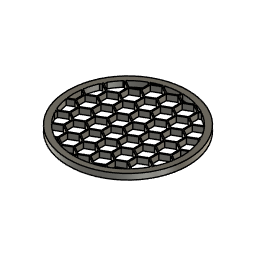
thermal_protection (Autodesk Fusion 360 design; units mm, degrees)
Autodesk Fusion 360 part; units mm, degrees
sketch "Sketch1" plane through (0, 0, 0) normal (0, 0, 1) x (1, 0, 0)
  circle A0 centre (0, 0) radius 21
  line L0 (0, -1.6166) -> (0, 1.6166)
  line L1 (0, 1.6166) -> (-2.8, 3.2332)
  line L2 (-2.8, 3.2332) -> (-5.6, 1.6166)
  line L3 (-5.6, 1.6166) -> (-5.6, -1.6166)
  line L4 (-5.6, -1.6166) -> (-2.8, -3.2332)
  line L5 (-2.8, -3.2332) -> (0, -1.6166)
  line L6 (5.6, -1.6166) -> (5.6, 1.6166)
  line L7 (5.6, 1.6166) -> (2.8, 3.2332)
  line L8 (2.8, 3.2332) -> (0, 1.6166)
  line L9 (0, 1.6166) -> (0, -1.6166)
  line L10 (0, -1.6166) -> (2.8, -3.2332)
  line L11 (2.8, -3.2332) -> (5.6, -1.6166)
  line L12 (-2.8, 0) -> (0, 0) construction
  line L13 (-2.8, 0) -> (-1.4, 2.4249) construction
  point P0 (-2.8, 0)
  point P1 (2.8, 0)
  dimension "d5" = 42
  dimension "d6" = 5.6
  constraint coincident A0.centre L12.end
  constraint vertical L3
  constraint vertical L0
  constraint coincident A0.centre L0
  constraint midpoint A0.centre L0
  constraint parallel L0 L9
  constraint coincident L0.end L1.start
  constraint coincident L0.start L5.end
  constraint coincident P0 L12.start
  constraint midpoint L1 L13.end
  measures "d5" diameter of A0
  measures "d6" distance of L0 L3
extrude "Extrude3" add sketch "Sketch1" along normal blind 2 thin wall 0.2 inside contours L0 L1 L2 L3 L4 L5 L9
extrude "Extrude4" add sketch "Sketch1" along normal up to surface (2 mm away) thin wall 0.2 inside contours L0 L6 L7 L8 L9 L10 L11
pattern_linear "R-Pattern2" count 14 spacing 5.6 along (1, 0, 0) both ways count 12 spacing 5.6 along (0.5, 0.866025, 0) both ways of "Extrude4"
extrude "Extrude5" cut sketch "Sketch1" along normal up to surface (2 mm away) contours A0 | L0 L1 L2 L3 L4 L5 L9 | L0 L6 L7 L8 L9 L10 L11 keep common part
extrude "Extrude6" add sketch "Sketch1" along normal up to surface (2 mm away) thin wall 2 inside contours A0 | L0 L1 L2 L3 L4 L5 L9 | L0 L6 L7 L8 L9 L10 L11
equation "OD = 42 mm"
equation "wall = 0.4 mm"
equation "owall = 2 mm"
equation "hsize = 5.2 mm + wall"
equation "d5 = OD"
equation "d6 = hsize"
equation "d17 = wall / 2"
equation "d18 = height"
equation "d20 = wall / 2"
equation "d25 = hsize"
equation "d26 = hsize"
equation "d29 = owall"
equation "height = 2 mm"
named bodies: "thermal_prot"
